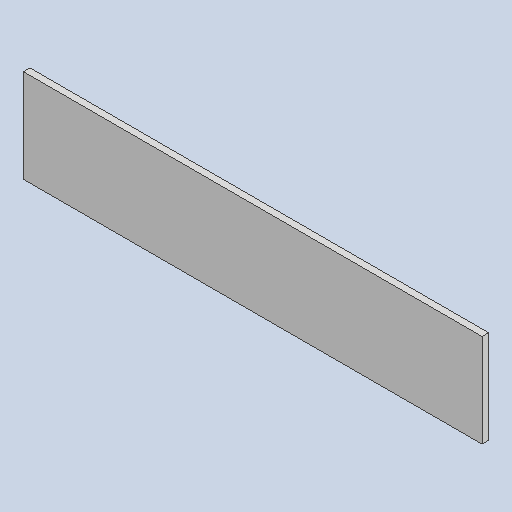
# Autodesk Inventor part: фанера_электр
Saved by Autodesk Inventor 2023.1 (Build 271208000, 208)
## iProperties
Created: 2025-12-30
Part Number: фанера_электр
Material: Типовые
Document SubType Name: Modeling
Designer: DELL
Density: 1 g/cm^3
Appearance: По умолчанию
Author: DELL
Autodesk Inventor part; units mm, degrees
ref_plane "YZ Plane" through (0, 0, 0) normal (1, 0, 0) x (0, 1, 0)
ref_plane "XZ Plane" through (0, 0, 0) normal (0, 1, 0) x (-1, 0, 0)
ref_plane "XY Plane" through (0, 0, 0) normal (0, 0, 1) x (1, 0, 0)
sketch "Эскиз1" plane through (0, 0, 0) normal (0, 0, 1) x (1, 0, 0)
  line L0 (-16.3474, 19.4) -> (16.3474, 19.4) projected
  line L1 (-30, 53.7) -> (-30, -13.3) projected
  line L2 (250.5, 53.7) -> (250.5, -13.3) projected
  line L3 (236.8474, 19.3225) -> (204.1526, 19.3225) projected
  line L4 (250.5, 19.4) -> (-30, 19.4)
  line L5 (-30, 19.4) -> (-30, -37.6)
  line L6 (-30, -37.6) -> (250.5, -37.6)
  line L7 (250.5, -37.6) -> (250.5, 19.4)
  point P0 (0, 0)
  point P1 (-30, 19.4)
  dimension "d0" = 280.5
  dimension "d1" = 57
  constraints: 8 end point, 2 parallel, 2 point on line, 1 horizontal, 1 perpendicular
  measures "d0" distance of L6.end L5.end
  measures "d1" distance of L5.end L4.end
extrude "Выдавливание1" add sketch "Эскиз1" along normal blind 4
